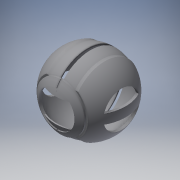
# Autodesk Inventor part: Wheatly
Saved by Autodesk Inventor 2019 (Build 230136000, 136)
## iProperties
Created: 2019-03-04
Part Number: Wheatly
Material: Generic
Document SubType Name: Modeling
Designer: 232963
Density: 1 g/cm^3
Appearance: Default
Author: 232963
Autodesk Inventor part; units mm, degrees
sketch "Sketch1" plane through (0, 0, 0) normal (0, 0, 1) x (1, 0, 0)
  arc A0 (0, -76.2) -> (0, 76.2) centre (0, 0) ccw
  line L0 (0, 89.4474) -> (0, -104.0758)
  dimension "d0" = 152.4
  constraints: 2 end point, 2 point on circle, 2 point on line, 1 centre point, 1 coincident, 1 vertical
  measures "d0" diameter of A0
revolve "Revolution1" add sketch "Sketch1" angle 360 about axis through (0, 89.4474, 0) along (0, -1, 0)
ref_plane "Work Plane1" through (0, 0, 76.2) normal (0, 0, 1) x (1, 0, 0)
sketch "Sketch2" plane through (0, 0, 76.2) normal (0, 0, 1) x (1, 0, 0)
  circle A0 centre (0, 0) radius 76.2 projected
  line L0 (-28.3981, 25.4) -> (28.3981, 25.4)
  line L1 (28.3981, -25.4) -> (-28.3981, -25.4)
  arc A1 (28.3981, -25.4) -> (28.3981, 25.4) centre (0, 0) ccw
  arc A2 (-28.3981, 25.4) -> (-28.3981, -25.4) centre (0, 0) ccw
  dimension "d5" = 25.4
  constraints: 4 end point, 4 point on circle, 2 centre point, 1 coincident, 1 horizontal, 1 parallel
  measures "d5" distance from line of point (0, 0) L0
extrude "Extrusion1" cut sketch "Sketch2" against normal blind 41.275 contours L0 A1 L1 A2
shell "Shell2" thickness 5.08 removed faces 1 at (-9.466, 8.4667, 34.925)
ref_plane "Work Plane2" through (0, 0, 69.85) normal (0, 0, 1) x (1, 0, 0)
sketch "Sketch3" plane through (0, 0, 69.85) normal (0, 0, 1) x (1, 0, 0)
  circle A0 centre (0, 0) radius 38.1
  circle A1 centre (0, 0) radius 50.8
  dimension "d13" = 76.2
  dimension "d14" = 101.6
  constraints: 2 centre point, 2 coincident
  measures "d13" diameter of A0
  measures "d14" diameter of A1
extrude "Extrusion2" add sketch "Sketch3" against normal blind 28.575
chamfer "Chamfer1" distance 12.7 angle 37 1 edges at (-50.8, 0, 69.85) measured on face at (-50.3, 0, 69.85)
ref_plane "Work Plane3" through (80.01, 0, 0) normal (1, 0, 0) x (0, 1, 0)
sketch "Sketch4" plane through (80.01, 0, 0) normal (1, 0, 0) x (0, 1, 0)
  arc A0 (-42.8048, 56.7961) -> (42.8048, 56.7961) centre (0, 0) ccw
  line L0 (-50.8, 56.7961) -> (50.8, 56.7961) projected
  constraints: 2 point on circle, 2 point on line, 1 centre point, 1 coincident
extrude "Extrusion3" add sketch "Sketch4" against normal blind 61.9125
sketch "Sketch5" plane through (0, 0, 76.2) normal (0, 0, 1) x (1, 0, 0)
  circle A0 centre (0, 0) radius 38.1 projected
  line L0 (-28.3981, -25.4) -> (28.3981, -25.4) projected
  line L1 (28.3981, 25.4) -> (-28.3981, 25.4) projected
  line L2 (28.3981, -25.4) -> (-28.3981, -25.4)
  line L3 (-28.3981, 25.4) -> (28.3981, 25.4)
  arc A1 (-28.3981, 25.4) -> (-28.3981, -25.4) centre (0, 0) ccw
  arc A2 (28.3981, -25.4) -> (28.3981, 25.4) centre (0, 0) ccw
  constraints: 5 end point, 4 point on circle, 2 centre point, 1 coincident, 1 horizontal, 1 parallel
extrude "Extrusion4" cut sketch "Sketch5" against normal blind 38.1 contours A0 L0 L1
sketch "Sketch6" plane through (0, 0, 38.1) normal (0, 0, 1) x (1, 0, 0)
  line L0 (18.0975, -25.4) -> (18.0975, 25.4) projected
  line L1 (18.0975, -25.4) -> (18.0975, 25.4) projected
  line L2 (28.3981, -25.4) -> (18.0975, -25.4) projected
  arc A0 (28.3981, -25.4) -> (28.3981, 25.4) centre (0, 0) ccw projected
  line L3 (18.0975, 25.4) -> (28.3981, 25.4) projected
extrude "Extrusion5" cut sketch "Sketch6" against normal blind 100.0125
sketch "Sketch7" plane through (0, 0, 0) normal (0, 0, 1) x (1, 0, 0)
  arc A0 (0, 78.74) -> (0, -78.74) centre (0, 0) ccw
  line L0 (0, -94.3931) -> (0, 121.4304)
  arc A1 (0, 109.8757) -> (0, -109.8757) centre (0, 0) ccw
  line L1 (0, -87.9915) -> (0, -163.9684)
  dimension "d27" = 78.74
  constraints: 5 point on line, 4 end point, 4 point on circle, 2 centre point, 2 vertical, 1 coincident
  measures "d27" radius of A0
revolve "Revolution2" cut sketch "Sketch7" angle 360 about axis through (0, -94.3931, 0) along (0, 1, 0) contours A0 L0 L1 A1
mirror "Mirror1" about plane through (0, 0, 0) normal (1, 0, 0) of "Extrusion3"
mirror "Mirror2" about plane through (0, 0, 0) normal (1, 0, 0) of "Revolution2"
sketch "Sketch8" plane through (0, 0, 76.2) normal (0, 0, 1) x (1, 0, 0)
  arc A0 (-28.3981, 25.4) -> (-28.3981, -25.4) centre (0, 0) ccw projected
  arc A1 (28.3981, 25.4) -> (-28.3981, 25.4) centre (0, 0) ccw projected
  line L0 (-28.3981, 25.4) -> (28.3981, 25.4)
  line L1 (-28.3981, -25.4) -> (28.3981, -25.4) projected
  line L2 (-28.3981, -25.4) -> (28.3981, -25.4)
  arc A2 (28.3981, -25.4) -> (28.3981, 25.4) centre (0, 0) ccw
  arc A3 (-28.3981, 25.4) -> (-28.3981, -25.4) centre (0, 0) ccw
  constraints: 4 end point, 4 point on circle, 2 centre point, 1 coincident, 1 collinear, 1 horizontal
extrude "Extrusion6" cut sketch "Sketch8" against normal blind 128.5875 contours L0 A2 L1 A0
ref_plane "Work Plane4" through (76.2, 0, 0) normal (1, 0, 0) x (0, 1, 0)
ref_plane "Work Plane5" through (-79.375, 0, 0) normal (1, 0, 0) x (0, 1, 0)
sketch "Sketch11" plane through (-79.375, 0, 0) normal (1, 0, 0) x (0, 1, 0)
  line L0 (-10.16, 42.7776) -> (10.16, 42.7776)
  line L1 (10.16, 42.7776) -> (10.16, -46.6665)
  line L2 (10.16, -46.6665) -> (-10.16, -46.6665)
  line L3 (-10.16, -46.6665) -> (-10.16, 42.7776)
  line L4 (0, 92.0235) -> (0, -69.7814) projected
  arc A0 (-10.16, 36.7204) -> (-10.16, -36.7204) centre (0, 0) ccw
  arc A1 (10.16, -36.7204) -> (10.16, 36.7204) centre (0, 0) ccw
  dimension "d34" = 10.16
  dimension "d35" = 20.32
  constraints: 8 end point, 4 point on circle, 4 point on line, 2 centre point, 2 parallel, 1 coincident, 1 horizontal, 1 perpendicular
  measures "d34" distance between parallel lines of L4 L3
  measures "d35" distance between parallel lines of L1 L3
extrude "Extrusion7" cut sketch "Sketch11" along normal blind 46.0375 contours L3 A0 | A1 L1
mirror "Mirror3" about plane through (0, 0, 0) normal (1, 0, 0) of "Extrusion7"
sketch "Sketch12" plane through (0, 0, 0) normal (0, 0, 1) x (1, 0, 0)
  line L0 (94.4392, 0) -> (-138.5212, 0)
  arc A0 (-73.66, 0) -> (73.66, 0) centre (0, 0) ccw
  point P0 (66.675, 0)
  point P1 (-66.675, 0)
  dimension "d39" = 147.32
  constraints: 4 point on line, 2 end point, 2 point on circle, 1 centre point, 1 horizontal
  measures "d39" diameter of A0
revolve "Revolution3" cut sketch "Sketch12" angle 360 about axis through (94.4392, 0, 0) along (-1, 0, 0)
sketch "Sketch13" plane through (80.01, 0, 0) normal (1, 0, 0) x (0, 1, 0)
  line L0 (-10.16, -36.7204) -> (-10.16, 36.7204) projected
  circle A0 centre (0, 0) radius 38.1
  constraints: 1 coincident, 3 other
sketch "Sketch14" plane through (0, 0, 0) normal (1, 0, 0) x (0, 1, 0)
  line L0 (38.1, 68.9085) -> (-38.1, 68.9085) projected
  line L1 (-38.1, 68.9085) -> (0, 0)
  constraints: 2 end point
sketch "Sketch18" plane through (0, 0, 0) normal (0, 0, 1) x (1, 0, 0)
  line L0 (-13.1237, 0) -> (26.9628, 0)
  point P0 (0, 0)
  constraints: 2 end point, 1 horizontal
ref_plane "Work Plane7" through (-13.1237, 0, 0) normal (0, -0.8751394, -0.483871) x (1, 0, 0)
sketch "Sketch19" plane through (-13.1237, 0, 0) normal (0, -0.8751394, -0.483871) x (1, 0, 0)
  circle A0 centre (13.1237, 0) radius 76.1869
  ellipse E0 centre (13.1237, 57.7514) end of major axis (-24.9763, 57.7514) minor radius 18.4355 (41.5218, 70.0418) -> (-15.2744, 70.0418) ccw projected
  line L0 (13.7587, 79.4645) -> (12.4887, 79.4645)
  line L1 (12.4887, 79.4645) -> (12.4887, 76.1843)
  line L2 (13.7587, 76.1843) -> (13.7587, 79.4645)
  line L3 (13.1237, 78.74) -> (13.1237, 0) projected
  line L4 (20.7269, 0) -> (-6.1377, 0)
  dimension "d49" = 1.27
  dimension "d50" = 0.635
  constraints: 8 end point, 2 horizontal, 2 point on circle, 1 centre point, 1 coincident, 1 parallel, 1 perpendicular, 2 other
  measures "d49" distance of L0.start L0.end
  measures "d50" distance between parallel lines of L3 L1
revolve "Revolution5" cut sketch "Sketch19" angle 360 about axis through (7.6032, 0, 0) along (-1, 0, 0) contours A0 L1 L0 L2
sketch "Sketch20" plane through (0, 0, 0) normal (1, 0, 0) x (0, 1, 0)
  arc A0 (-50.796, 56.7961) -> (50.796, 56.7961) centre (0, 0) ccw projected
  line L0 (-50.796, 56.7961) -> (0, 0)
  line L1 (0, 101.4466) -> (0, -105.8047) projected
  dimension "d52" = 41.808
  constraints: 2 end point
  measures "d52" angle of L1 L0
ref_plane "Work Plane8" through (0, -50.796, 56.7961) normal (0, 0.7453819, 0.6666377) x (0, 0.6666377, -0.7453819)
sketch "Sketch21" plane through (0, -50.796, 56.7961) normal (0, 0.7453819, 0.6666377) x (0, 0.6666377, -0.7453819)
  ellipse E0 centre (93.13, 0) end of major axis (93.13, 71.8282) minor radius 53.5394 (39.5926, 0.635) -> (39.5926, -0.635) ccw projected
  line L0 (5.7274, -0.635) -> (39.5926, -0.635) projected
  ellipse E1 centre (59.2648, 0) end of major axis (59.2648, 71.8282) minor radius 53.5394 (5.7274, 0.635) -> (5.7274, -0.635) ccw projected
  line L1 (5.7274, 0.635) -> (39.5926, 0.635) projected
  circle A0 centre (76.1974, 0) radius 76.2
  line L2 (0.0635, 3.175) -> (2.794, 3.175)
  line L3 (2.794, 3.175) -> (2.794, -3.175)
  line L4 (2.794, -3.175) -> (0.0635, -3.175)
  line L5 (0, 0) -> (76.1974, 0) projected
  line L6 (-0.8472, -0.635) -> (-0.8472, 0)
  line L7 (-0.8472, 0.635) -> (-0.8472, 1.905)
  line L8 (76.1974, -20.818) -> (76.1974, 9.8053)
  dimension "d53" = 152.4
  dimension "d54" = 2.54
  dimension "d55" = 3.175
  dimension "d56" = 2.794
  dimension "d58" = 6.35
  constraints: 12 end point, 3 parallel, 3 point on line, 2 point on circle, 1 centre point, 1 coincident, 1 horizontal, 1 perpendicular, 1 vertical, 2 other
  measures "d53" diameter of A0
  measures "d54" distance of L6.start L7.end
  measures "d55" distance between parallel lines of L5 L4
  measures "d56" distance from line of L5.start L3
  measures "d58" distance of L2.end L3.end
revolve "Revolution6" cut sketch "Sketch21" angle 276.38 about axis through (20.818, 0, 0) along (1, 0, 0) picked at (1.8643, -1.4112) contours L2 L3 L4 A0
body "Solid1"
